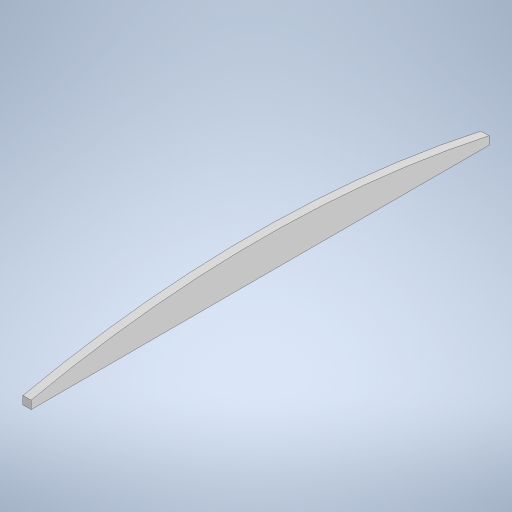
# Autodesk Inventor part: shorthalfofSidestrip_Ocampo
Saved by Autodesk Inventor 2023 (Build 270158000, 158)
## iProperties
Created: 2025-03-25
Part Number: shorthalfofSidestrip_Ocampo
Material: Generic
Document SubType Name: Modeling
Designer: 1244275
Density: 1 g/cm^3
Appearance: Default
Author: 1244275
Autodesk Inventor part; units mm, degrees
ref_plane "YZ Plane" through (0, 0, 0) normal (1, 0, 0) x (0, 1, 0)
ref_plane "XZ Plane" through (0, 0, 0) normal (0, 1, 0) x (-1, 0, 0)
ref_plane "XY Plane" through (0, 0, 0) normal (0, 0, 1) x (1, 0, 0)
sketch "Sketch1" plane through (0, 0, 0) normal (1, 0, 0) x (0, 1, 0)
  line L0 (0, 0) -> (0, -355.8794)
  line L1 (0, 0) -> (6.35, 0)
  line L2 (0, -355.8794) -> (6.35, -355.8794)
  arc A0 (6.35, -355.8794) -> (6.35, 0) centre (-804.101, -177.9397) ccw
  dimension "d0" = 355.8794
  dimension "d1" = 6.35
  dimension "d2" = 6.35
  constraints: 6 end point, 2 horizontal, 2 point on circle, 1 centre point, 1 vertical
  measures "d0" distance of L0.start L0.end
  measures "d1" distance of L0.start L1.end
  measures "d2" distance of L0.end L2.end
extrude "Extrusion1" add sketch "Sketch1" along normal blind 6.35
body "Solid1"
